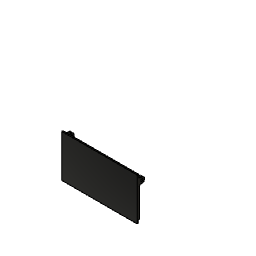
Abdeckung_hinten_v56 (Autodesk Fusion 360 design; units mm, degrees)
Autodesk Fusion 360 part; units mm, degrees
note: some values were not read from the file. Chosen so that the rebuilt part matches the saved one: which pieces of a blend or face edit are solid.
sketch "Skizze1" plane through (0, 0, 0) normal (1, 0, 0) x (0, 1, 0)
  line L0 (-75, -0.2) -> (-75, 5.1)
  line L1 (-74.1, 5.1) -> (-75, 5.1)
  line L2 (-74.1, 71.3) -> (-73.2, 71.3)
  line L3 (-74.1, 77.1) -> (-74.1, 71.3)
  line L4 (-75, 5.1) -> (-72.8, 5.1)
  line L5 (-75, 5.1) -> (-75, -0.2)
  line L6 (-75, -0.2) -> (-76.5, -0.2)
  line L7 (-76.5, -0.2) -> (-76.5, 77.1)
  line L8 (-76.5, 77.1) -> (-74.1, 77.1)
  line L9 (-74.1, 77.1) -> (-74.1, 71.3)
  line L10 (-72.8, 5.1) -> (-72.8, 71.3)
  line L11 (-74.1, 71.3) -> (-72.8, 71.3)
  dimension "d181" = 2.2
  dimension "d182" = 1.5
  constraint coincident L0.end L1.end
  constraint perpendicular L0 L4
  constraint coincident L0.start L5.end
  constraint perpendicular L5 L6
  constraint perpendicular L6 L7
  constraint coincident L3.start L8.end
  constraint coincident L2.start L3.end
  constraint horizontal L8
  constraint perpendicular L4 L10
  constraint horizontal L11
  measures "d181" distance of L0.end L4.end
  measures "d182" distance of L0.start L6.end
extrude "Extrusion1" add sketch "Skizze1" along normal mid plane 138.2
sketch "Skizze2" plane through (0, 0, 10.5) normal (0, 0, 1) x (-1, 0, 0)
  circle A0 centre (-33.9, 67.5) radius 1.9
  circle A1 centre (-33.9, -67.5) radius 1.9
  circle A2 centre (61.1, -67.5) radius 1.9
  circle A3 centre (61.1, 67.5) radius 1.9
  circle A4 centre (50.1, -64.7) radius 6.6
  circle A5 centre (20.6, -66.2) radius 5.1
  line L0 (68.1, -72.5) -> (68.1, 72.5)
  line L1 (68.1, 72.5) -> (-42.9, 72.5)
  line L2 (-42.9, 72.5) -> (-42.9, -72.5)
  line L3 (-42.9, -72.5) -> (68.1, -72.5)
  line L4 (69.1, 72.8) -> (-69.1, 72.8)
  line L5 (64.85, 67.5) -> (64.85, 72.8)
  line L6 (57.35, 67.5) -> (57.35, 72.8)
  arc A6 (57.35, 67.5) -> (64.85, 67.5) centre (61.1, 67.5) ccw
  line L7 (-30.15, 67.5) -> (-30.15, 72.8)
  line L8 (-37.65, 67.5) -> (-37.65, 72.8)
  arc A7 (-37.65, 67.5) -> (-30.15, 67.5) centre (-33.9, 67.5) ccw
  dimension "d186" = 7.5
  dimension "d187" = 7.5
  constraint concentric A3 A6
  constraint coincident L4 L5.end
  constraint coincident L4 L6.end
  constraint tangent L6 A6
  constraint tangent L5 A6
  constraint vertical L5
  constraint vertical L6
  constraint concentric A0 A7
  constraint coincident L4 L7.end
  constraint perpendicular L4 L7
  constraint coincident L4 L8.end
  constraint perpendicular L4 L8
  constraint tangent L8 A7
  constraint tangent L7 A7
  measures "d186" diameter of A6
  measures "d187" diameter of A7
extrude "Extrusion2" add sketch "Skizze2" along normal blind 2 contours L1 L5 L6 A6 | L1 L4 L5 L6 | L1 L4 L7 L8 | L1 L7 L8 A7
sketch "Skizze4" plane through (-69.1, 0, 2) normal (1, 0, 0) x (0, 1, 0)
  circle A0 centre (63.2, 63.1) radius 1.5
  circle A1 centre (-63.2, 63.1) radius 1.5
  line L0 (73.2, 81.3) -> (-73.2, 81.3)
  line L1 (-73.2, 81.3) -> (-73.2, -0.2)
  line L2 (-73.2, -0.2) -> (73.2, -0.2)
  line L3 (73.2, -0.2) -> (73.2, 81.3)
  line L4 (-72.8, 71.3) -> (-72.8, 5.1)
  line L5 (-63.2, 68.1) -> (-72.8, 68.1)
  line L6 (-63.2, 58.1) -> (-72.8, 58.1)
  arc A2 (-63.2, 58.1) -> (-63.2, 68.1) centre (-63.2, 63.1) ccw
  circle A3 centre (-63.2, 63.1) radius 2.1
  dimension "d204" = 10
  dimension "d1065" = 4.2
  constraint concentric A1 A2
  constraint coincident L4 L5.end
  constraint perpendicular L4 L5
  constraint coincident L4 L6.end
  constraint tangent L6 A2
  constraint tangent L5 A2
  constraint perpendicular L4 L6
  constraint concentric A2 A3
  measures "d204" diameter of A2
  measures "d1065" diameter of A3
extrude "Extrusion3" add sketch "Skizze4" along normal blind 4.5 contours L4 L5 L6 A2
sketch "Skizze5" plane through (69.1, 0, 2) normal (-1, 0, 0) x (0, -1, 0)
  circle A0 centre (68.2, 63.1) radius 1.5
  circle A1 centre (-63.2, 48.1) radius 1.5
  line L0 (73.2, 81.3) -> (-73.2, 81.3)
  line L1 (-73.2, 81.3) -> (-73.2, -0.2)
  line L2 (-73.2, -0.2) -> (73.2, -0.2)
  line L3 (73.2, -0.2) -> (73.2, 81.3)
  line L4 (72.8, 5.1) -> (72.8, 71.3)
  line L5 (68.2, 68.1) -> (72.8, 68.1)
  line L6 (68.2, 58.1) -> (72.8, 58.1)
  arc A2 (68.2, 68.1) -> (68.2, 58.1) centre (68.2, 63.1) ccw
  circle A3 centre (68.2, 63.1) radius 2.1
  dimension "d207" = 10
  dimension "d1064" = 4.2
  constraint concentric A0 A2
  constraint coincident L4 L5.end
  constraint perpendicular L4 L5
  constraint coincident L4 L6.end
  constraint perpendicular L4 L6
  constraint tangent L6 A2
  constraint tangent L5 A2
  constraint concentric A2 A3
  measures "d207" diameter of A2
  measures "d1064" diameter of A3
extrude "Extrusion4" add sketch "Skizze5" along normal blind 4.5 contours L4 L5 L6 A2
fillet "Abrundung2" radius 3 12 edges at (33.9, -72.8, 12.5) (37.65, -72.8, 11.5) (30.15, -72.8, 11.5) (-61.1, -72.8, 12.5) (-64.85, -72.8, 11.5) (-57.35, -72.8, 11.5) (66.85, -72.8, 70.1) (66.85, -72.8, 60.1) (64.6, -72.8, 65.1) (-66.85, -72.8, 70.1) (-64.6, -72.8, 65.1) (-66.85, -72.8, 60.1)
